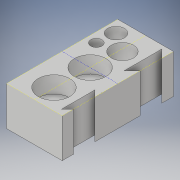
# Autodesk Inventor part: last_drill
Saved by Autodesk Inventor 2019 (Build 230136000, 136)
## iProperties
Created: 2018-12-20
Part Number: last_drill
Material: Generic
Document SubType Name: Modeling
Designer: assman
Density: 1 g/cm^3
Appearance: Default
Author: assman
## iProperties of the stored document last_drill_3DPrint.ipt
Created: 2018-12-20
Part Number: last_drill_3DPrint
Material: Generic
Document SubType Name: Modeling
Designer: assman
Density: 1 g/cm^3
Appearance: Default
Author: assman
Autodesk Inventor part; units mm, degrees
ref_plane "YZ Plane" through (0, 0, 0) normal (1, 0, 0) x (0, 1, 0)
ref_plane "XZ Plane" through (0, 0, 0) normal (0, 1, 0) x (-1, 0, 0)
ref_plane "XY Plane" through (0, 0, 0) normal (0, 0, 1) x (1, 0, 0)
sketch "Sketch1" plane through (0, 0, 0) normal (0, 1, 0) x (-1, 0, 0)
  line L0 (0, 0) -> (10, 0)
  line L1 (10, 0) -> (10, -20)
  line L2 (10, -20) -> (0, -20)
  line L3 (0, -20) -> (0, 0)
  dimension "d0" = 10
  dimension "d1" = 20
  constraints: 8 end point, 2 parallel, 1 coincident, 1 horizontal, 1 perpendicular
  measures "d0" distance of L1.end L2.end
  measures "d1" distance of L0.end L1.end
extrude "Extrusion1" add sketch "Sketch1" along normal blind 7
sketch "Sketch2" plane through (0, 7, 0) normal (0, 1, 0) x (1, 0, 0)
  line L0 (-10, 20) -> (-10, 0) construction
  line L1 (-5, 20) -> (-5, 0) construction
  line L2 (-10, 0) -> (0, 0) construction
  line L3 (-10, 10) -> (0, 10) construction
  line L4 (0, 0) -> (0, 20) construction
  constraints: 4 end point, 3 midpoint
sketch "Sketch3" plane through (0, 7, 0) normal (0, 1, 0) x (1, 0, 0)
  point P0 (0, 0)
  point P1 (-5.1203, 3.6397)
hole "Hole1" at (-5.1203, 7, -3.6397) direction (0, -1, 0) diameter 2.85 depth 13.15 counterbore diameter 5.65 counterbore depth 3
sketch "Sketch4" plane through (0, 7, 0) normal (0, 1, 0) x (1, 0, 0)
  point P0 (0, 0)
  point P1 (-4.9804, 10.0094)
hole "Hole2" at (-4.9804, 7, -10.0094) direction (0, -1, 0) diameter 2.85 depth 9.05 counterbore diameter 5.65 counterbore depth 3
sketch "Sketch5" plane through (0, 7, 0) normal (0, 1, 0) x (1, 0, 0)
  point P0 (0, 0)
  point P1 (-8.0124, 17.6811)
hole "Hole3" at (-8.0124, 7, -17.6811) direction (0, -1, 0) diameter 3 end through all
sketch "Sketch6" plane through (0, 7, 0) normal (0, 1, 0) x (1, 0, 0)
  point P0 (0, 0)
  point P1 (-8.2667, 14.4)
hole "Hole4" at (-8.2667, 7, -14.4) direction (0, -1, 0) diameter 2 end through all
sketch "Sketch7" plane through (0, 7, 0) normal (0, 1, 0) x (1, 0, 0)
  point P0 (0, 0)
  point P1 (-4.5699, 15.3923)
hole "Hole5" at (-4.5699, 7, -15.3923) direction (0, -1, 0) diameter 4 end through all
sketch "Sketch8" plane through (0, 7, 0) normal (0, 1, 0) x (1, 0, 0)
  line L0 (0, 0) -> (0, 20) projected
  line L1 (0, 14.0043) -> (-1.4223, 12.582)
  line L2 (-1.4223, 12.582) -> (-1.4223, 19.3282)
  line L3 (-1.4223, 19.3282) -> (0, 17.9058)
  line L4 (0, 14.0043) -> (0, 17.9058)
  dimension "d39" = 45
  dimension "d40" = 45
  dimension "d41" = 6.7462
  dimension "d42" = 1.4223
  constraints: 8 end point, 2 point on line, 1 collinear, 1 parallel
  measures "d39" angle of L0 L1
  measures "d40" angle of L0 L3
  measures "d41" distance of L1.end L2.end
  measures "d42" distance between parallel lines of L0 L2
extrude "Extrusion2" cut sketch "Sketch8" against normal through all
sketch "Sketch9" plane through (0, 7, 0) normal (0, 1, 0) x (1, 0, 0)
  line L0 (0, 14.0043) -> (0, 0) projected
  line L1 (0, 2.0269) -> (-1.0707, 0.9562)
  line L2 (-1.0707, 0.9562) -> (-1.0707, 6.9582)
  line L3 (-1.0707, 6.9582) -> (0, 5.8875)
  dimension "d45" = 45
  dimension "d46" = 45
  dimension "d47" = 6.002
  dimension "d48" = 1.0707
  constraints: 6 end point, 2 point on line, 1 parallel
  measures "d45" angle of L0 L1
  measures "d46" angle of L0 L3
  measures "d47" distance of L1.end L2.end
  measures "d48" distance between parallel lines of L0 L2
extrude "Extrusion3" cut sketch "Sketch9" against normal blind 7
equation "\"d40\" = d39"
equation "\"d46\" = d45"
body "Solid1"
